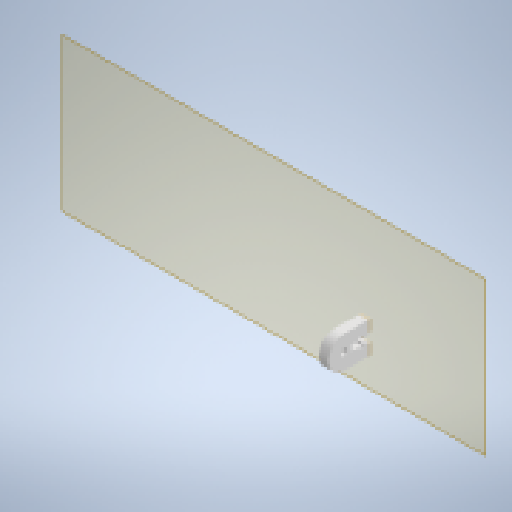
# Autodesk Inventor part: Крепление рычага к лицу
Saved by Autodesk Inventor 2023.2 (Build 272271030, 271C)
## iProperties
Created: 2024-02-06
Part Number: Крепление рычага к лицу
Material: Типовые
Document SubType Name: Modeling
Designer: I9232
Density: 1 g/cm^3
Appearance: По умолчанию
Author: I9232
Autodesk Inventor part; units mm, degrees
ref_plane "YZ Plane" through (0, 0, 0) normal (1, 0, 0) x (0, 1, 0)
ref_plane "XZ Plane" through (0, 0, 0) normal (0, 1, 0) x (-1, 0, 0)
ref_plane "XY Plane" through (0, 0, 0) normal (0, 0, 1) x (1, 0, 0)
sketch "Эскиз1" plane through (0, 0, 0) normal (0, 0, 1) x (1, 0, 0)
  line L0 (59.1195, 52.8794) -> (53.1195, 52.8794)
  line L1 (53.1195, 52.8794) -> (53.1195, 72.8794)
  line L2 (53.1195, 72.8794) -> (59.1195, 72.8794)
  line L3 (59.1195, 72.8794) -> (59.1195, 52.8794)
  point P0 (0, 0)
  dimension "d0" = 20
  dimension "d1" = 6
  constraints: 8 end point, 2 parallel, 1 horizontal, 1 perpendicular
  measures "d0" distance of L0.end L1.end
  measures "d1" distance of L1.end L2.end
extrude "Выдавливание1" add sketch "Эскиз1" along normal blind 25
fillet "Сопряжение1" radius 10 2 edges at (56.1195, 52.8794, 25) (56.1195, 72.8794, 25)
sketch "Эскиз2" plane through (53.1195, 52.8794, 0) normal (-1, 0, 0) x (0, 0, 1)
  circle A0 centre (15, 10) radius 2
  line L0 (0, 20) -> (0, 0) projected
  line L1 (0, 10) -> (25, 10) construction
  arc A1 (15, 0) -> (15, 20) centre (15, 10) ccw projected
  point P0 (0, -52.8794)
  dimension "d5" = 4
  constraints: 2 end point, 1 centre point, 1 coincident, 1 horizontal, 1 midpoint, 1 point on circle
  measures "d5" diameter of A0
extrude "Выдавливание2" cut sketch "Эскиз2" against normal up to surface (6 mm away)
sketch "Эскиз3" plane through (0, 0, 0) normal (0, 0, -1) x (-1, 0, 0)
  line L0 (-53.1195, 52.8794) -> (-59.1195, 52.8794)
  line L1 (-59.1195, 52.8794) -> (-59.1195, 59.8794)
  line L2 (-59.1195, 59.8794) -> (-53.1195, 59.8794)
  line L3 (-53.1195, 59.8794) -> (-53.1195, 52.8794)
  line L4 (-59.1195, 72.8794) -> (-53.1195, 72.8794) projected
  line L5 (-59.1195, 72.8794) -> (-53.1195, 72.8794)
  line L6 (-53.1195, 72.8794) -> (-53.1195, 65.8794)
  line L7 (-53.1195, 65.8794) -> (-59.1195, 65.8794)
  line L8 (-59.1195, 65.8794) -> (-59.1195, 72.8794)
  point P0 (0, 0)
  dimension "d8" = 7
  dimension "d9" = 7
  dimension "d18" = 6
  constraints: 16 end point, 4 parallel, 2 horizontal, 2 perpendicular, 1 point on line
  measures "d8" distance of L0.end L1.end
  measures "d9" distance of L7.end L4.start
  measures "d18" distance of L0.start L0.end
extrude "Выдавливание3" add sketch "Эскиз3" along normal blind 2
sketch "Эскиз4" plane through (53.1195, 62.8794, 15) normal (-1, 0, 0) x (0, 0, 1)
  line L0 (-15, 3) -> (-15, -3) projected
  line L1 (-15, 0) -> (-4.7, 0)
  line L2 (-4.7, 0) -> (-4.7, -1.75)
  line L3 (-15, -1.75) -> (-15, 0)
  line L4 (-4.7, 0) -> (-4.7, 1.75)
  line L5 (-10.2565, 0) -> (-12.2169, 0)
  line L6 (-12.2169, -1.75) -> (-12.2169, -3.05)
  line L7 (-12.2169, -3.05) -> (-9.7169, -3.05)
  line L8 (-9.7169, -3.05) -> (-9.7169, -1.75)
  line L9 (-12.2169, 1.75) -> (-12.2169, 3.05)
  line L10 (-12.2169, 3.05) -> (-9.7169, 3.05)
  line L11 (-9.7169, 3.05) -> (-9.7169, 1.75)
  line L12 (-4.7, -1.75) -> (-9.7169, -1.75)
  line L13 (-12.2169, -1.75) -> (-15, -1.75)
  line L14 (-4.7, 1.75) -> (-9.7169, 1.75)
  line L15 (-12.2169, 1.75) -> (-15, 1.75)
  line L16 (-4.7, 1.75) -> (-9.7169, 1.75)
  line L17 (-12.2169, 1.75) -> (-15, 1.75)
  point P0 (-15, -62.8794)
  point P1 (-15, 1.75)
  point P2 (-15, -1.75)
  dimension "d12" = 10.3
  dimension "d13" = 1.75
  dimension "d16" = 2.5
  dimension "d17" = 6.1
  constraints: 34 end point, 5 parallel, 4 symmetric about line, 2 horizontal, 2 perpendicular, 1 midpoint, 1 point on line
  measures "d12" distance of L2.end L3.start
  measures "d13" distance of L1.end L2.end
  measures "d16" distance of L6.end L7.end
  measures "d17" distance of L11.start L7.end
extrude "Выдавливание4" cut sketch "Эскиз4" against normal up to surface (6 mm away)
